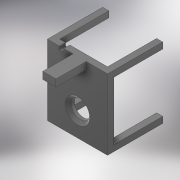
# Autodesk Inventor part: Senso_Halter
Saved by Autodesk Inventor 2020 (Build 240168000, 168)
## iProperties
Created: 2022-02-19
Part Number: Senso_Halter
Material: Acetalharz, Schwarz
Document SubType Name: Modeling
Designer: Julian Uhl
Density: 1.425 g/cm^3
Appearance: Glatt - Schwarz
Mass: 202.941 g
Surface Area: 425.299 cm^2
Volume: 142.415 cm^3
Author: Julian Uhl
Autodesk Inventor part; units mm, degrees
ref_plane "YZ Plane" through (0, 0, 0) normal (1, 0, 0) x (0, 1, 0)
ref_plane "XZ Plane" through (0, 0, 0) normal (0, 1, 0) x (-1, 0, 0)
ref_plane "XY Plane" through (0, 0, 0) normal (0, 0, 1) x (1, 0, 0)
sketch "Skizze1" plane through (0, 0, 0) normal (0, 0, 1) x (1, 0, 0)
  line L0 (-19.6, 0) -> (117.6, 0) projected
  line L1 (0, -23) -> (0, 138) projected
  line L2 (0, 0) -> (98, 0)
  line L3 (98, 0) -> (98, 115)
  line L4 (98, 115) -> (0, 115)
  line L5 (0, 115) -> (0, 0)
  point P0 (0, 115)
  dimension "d0" = 115
  dimension "d1" = 98
  constraints: 8 end point, 2 parallel, 1 horizontal, 1 perpendicular
  measures "d0" distance between parallel lines of L0 L4
  measures "d1" distance between parallel lines of L3 L1
extrude "Extrusion1" add sketch "Skizze1" along normal blind 10
sketch "Skizze2" plane through (0, 0, 10) normal (0, 0, 1) x (1, 0, 0)
  line L0 (98, 115) -> (0, 115) projected
  line L1 (41.65, 115) -> (63.15, 115)
  line L2 (63.15, 115) -> (63.15, 103.5)
  line L3 (63.15, 103.5) -> (41.65, 103.5)
  line L4 (41.65, 103.5) -> (41.65, 115)
  line L5 (98, 0) -> (98, 115) projected
  point P0 (0, 0)
  dimension "d4" = 21.5
  dimension "d5" = 11.5
  dimension "d6" = 34.85
  constraints: 8 end point, 2 parallel, 1 horizontal, 1 perpendicular, 1 point on line
  measures "d4" distance between parallel lines of L2 L4
  measures "d5" distance between parallel lines of L3 L0
  measures "d6" distance between parallel lines of L5 L2
extrude "Extrusion2" add sketch "Skizze2" along normal blind 49.2
sketch "Skizze3" plane through (41.65, 103.5, 10) normal (-1, 0, 0) x (0, 0, 1)
  line L0 (45.2, 7.5) -> (45.2, 4)
  line L1 (45.2, 4) -> (43.7, 4)
  line L2 (43.7, 4) -> (43.7, 2.8888)
  line L3 (0, 0) -> (0, 11.5) projected
  line L4 (45.2, 7.5) -> (0, 7.5)
  line L5 (0, 11.5) -> (0, 0) projected
  line L6 (0, 4) -> (0, 7.5)
  line L7 (49.2, 11.5) -> (49.2, 0) projected
  line L8 (0, 11.5) -> (49.2, 11.5) projected
  line L9 (0, 0) -> (49.2, 0) projected
  line L10 (1.5, 2.8888) -> (1.5, 4)
  line L11 (1.5, 4) -> (0, 4)
  line L12 (43.7, 2.8888) -> (43.7, 0)
  line L13 (1.5, 2.8888) -> (1.5, 0)
  point P0 (-10, -103.5)
  point P1 (0, 4)
  dimension "d9" = 4
  dimension "d10" = 4
  dimension "d11" = 4
  dimension "d12" = 4
  dimension "d13" = 1.5
  dimension "d14" = 1.5
  constraints: 18 end point, 5 perpendicular, 2 point on line, 2 vertical, 1 collinear
  measures "d9" distance between parallel lines of L7 L0
  measures "d10" distance between parallel lines of L8 L4
  measures "d11" distance between parallel lines of L9 L1
  measures "d12" distance between parallel lines of L9 L11
  measures "d13" distance between parallel lines of L2 L0
  measures "d14" distance between parallel lines of L3 L10
extrude "Extrusion3" cut sketch "Skizze3" against normal blind 17.5 contours L0 L1 L2 L12 L9 L13 L10 L11 L3 L4
sketch "Skizze4" plane through (0, 0, 10) normal (0, 0, 1) x (1, 0, 0)
  line L0 (98, 115) -> (0, 115) projected
  line L1 (19.65, 115) -> (26.65, 115)
  line L2 (26.65, 115) -> (26.65, 110)
  line L3 (26.65, 110) -> (19.65, 110)
  line L4 (19.65, 110) -> (19.65, 115)
  line L5 (41.65, 115) -> (41.65, 103.5) projected
  point P0 (0, 0)
  dimension "d17" = 7
  dimension "d18" = 5
  dimension "d19" = 15
  constraints: 8 end point, 2 parallel, 1 horizontal, 1 perpendicular, 1 point on line
  measures "d17" distance between parallel lines of L2 L4
  measures "d18" distance between parallel lines of L0 L3
  measures "d19" distance between parallel lines of L5 L2
extrude "Extrusion4" cut sketch "Skizze4" against normal blind 10
sketch "Skizze5" plane through (0, 0, 0) normal (0, 0, -1) x (-1, 0, 0)
  line L0 (-19.65, 115) -> (0, 115) projected
  line L1 (0, 115) -> (0, 0) projected
  line L2 (-10, 115) -> (0, 115)
  line L3 (0, 115) -> (0, 105)
  line L4 (0, 105) -> (-10, 105)
  line L5 (-10, 105) -> (-10, 115)
  line L6 (0, 0) -> (-98, 0) projected
  line L7 (0, 10) -> (-10, 10)
  line L8 (-10, 10) -> (-10, 0)
  line L9 (-10, 0) -> (0, 0)
  line L10 (0, 0) -> (0, 10)
  line L11 (-98, 10) -> (-88, 10)
  line L12 (-88, 10) -> (-88, 0)
  line L13 (-88, 0) -> (-98, 0)
  line L14 (-98, 0) -> (-98, 10)
  line L15 (-98, 115) -> (-26.65, 115) projected
  line L16 (-88, 115) -> (-98, 115)
  line L17 (-98, 115) -> (-98, 105)
  line L18 (-98, 105) -> (-88, 105)
  line L19 (-88, 105) -> (-88, 115)
  line L20 (-98, 0) -> (-98, 115) projected
  point P0 (-98, 0)
  point P1 (-88, 0)
  dimension "d22" = 10
  dimension "d23" = 10
  dimension "d24" = 10
  dimension "d25" = 10
  dimension "d26" = 10
  dimension "d27" = 10
  dimension "d28" = 10
  dimension "d29" = 10
  dimension "d40" = 0
  constraints: 32 end point, 8 parallel, 7 point on line, 4 horizontal, 4 perpendicular
  measures "d22" distance between parallel lines of L18 L16
  measures "d23" distance between parallel lines of L17 L19
  measures "d24" distance between parallel lines of L14 L12
  measures "d25" distance between parallel lines of L6 L11
  measures "d26" distance of L7.end L8.end
  measures "d27" distance between parallel lines of L8 L1
  measures "d28" distance between parallel lines of L1 L5
  measures "d29" distance between parallel lines of L0 L4
  measures "d40" distance between parallel lines of L20 L17
extrude "Extrusion5" add sketch "Skizze5" along normal blind 80
sketch "Skizze6" plane through (0, 0, 10) normal (0, 0, 1) x (1, 0, 0)
  circle A0 centre (49, 38.5) radius 15
  line L0 (0, 115) -> (0, 0) projected
  line L1 (41.65, 103.5) -> (63.15, 103.5) projected
  dimension "d32" = 30
  dimension "d33" = 49
  dimension "d34" = 65
  constraints: 1 centre point
  measures "d32" diameter of A0
  measures "d33" distance from line of L0 A0.centre
  measures "d34" distance from line of A0.centre L1
extrude "Extrusion6" cut sketch "Skizze6" against normal blind 10
chamfer "Fase1" distance 5 angle 45 1 edges at (34, 38.5, 10)
